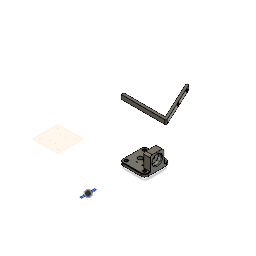
mangaScreenPostMount (Autodesk Fusion 360 design; units mm, degrees)
Autodesk Fusion 360 part; units mm, degrees
sketch "Sketch2" plane through (0, 0, 0) normal (0, 1, 0) x (1, 0, 0)
  circle A0 centre (0, -5) radius 20
  dimension "d26" = 40
  measures "d26" diameter of A0
sketch "Sketch3" plane through (0, 0, 0) normal (0, 1, 0) x (1, 0, 0)
  circle A0 centre (0.421, 74.5094) radius 20
  dimension "d29" = 40
  measures "d29" diameter of A0
sketch "Sketch4" plane through (0, 0, 0) normal (0, 1, 0) x (1, 0, 0)
sketch "Sketch5" plane through (0, 0, 0) normal (0, 1, 0) x (1, 0, 0)
  circle A0 centre (39.3711, 35) radius 20
  dimension "d32" = 40
  measures "d32" diameter of A0
sketch "Sketch6" plane through (0, 0, 0) normal (0, 1, 0) x (1, 0, 0)
sketch "Sketch7" plane through (0, 0, 0) normal (0, 1, 0) x (1, 0, 0)
sketch "Sketch8" plane through (0, 0, 0) normal (0, 1, 0) x (1, 0, 0)
sketch "Sketch9" plane through (0, 0, 0) normal (0, 1, 0) x (1, 0, 0)
sketch "Sketch11" plane through (0, 0, 0) normal (0, 1, 0) x (1, 0, 0)
  line L0 (-185, 0) -> (-64.7091, 0)
  line L1 (-61.9901, 4.2679) -> (-113.6725, 115.1011)
  line L2 (-117.6593, 116.5522) -> (-118.5656, 116.1295)
  line L3 (-185, 0) -> (-185, 5)
  line L4 (-182, 8) -> (-80, 8)
  line L5 (-120.0167, 112.1428) -> (-71.4609, 8.0146)
  line L6 (-80, 8) -> (-71.4609, 8.0146)
  arc A0 (-182, 8) -> (-185, 5) centre (-182, 5) ccw
  arc A1 (-118.5656, 116.1295) -> (-120.0167, 112.1428) centre (-117.2978, 113.4106) ccw
  arc A2 (-113.6725, 115.1011) -> (-117.6593, 116.5522) centre (-116.3914, 113.8332) ccw
  arc A3 (-64.7091, 0) -> (-61.9901, 4.2679) centre (-64.7091, 3) ccw
  dimension "d43" = 65
  dimension "d44" = 130
  dimension "d45" = 7
  dimension "d46" = 8
  dimension "d47" = 3
  dimension "d48" = 3
  dimension "d49" = 3
  dimension "d50" = 3
  measures "d43" angle of L0 L1
  measures "d46" distance of origin
  measures "d47" radius of A0
  measures "d48" radius of A1
  measures "d49" radius of A2
  measures "d50" radius of A3
extrude "Extrude4" add sketch "Sketch11" along normal blind 12 makes body 1
move_body "Move4" bodies 1 to x (1, 0, 0) y (0, 1, 0) z (0, 0, 1) at (70, 0, -150)
hole "Hole5" at (-39.4463, 6, -256.038) direction (-0.906308, 0, 0.422618) diameter 3.8 depth 8 tip angle 180 bodies 1
hole "Hole6" at (-39.4463, 6, -256.038) direction (-0.906308, 0, 0.422618) diameter 7.5 depth 2 tip angle 180 bodies 1
hole "Hole7" at (-45.7905, 6, -253.0797) direction (0.906308, 0, -0.422618) diameter 7.2 depth 4 tip angle 180 bodies 1
hole "Hole8" at (-18.3154, 6, -210.7226) direction (-0.906308, 0, 0.422618) diameter 3.8 depth 8 tip angle 180 bodies 1
hole "Hole9" at (-18.3154, 6, -210.7226) direction (-0.906308, 0, 0.422618) diameter 7.5 depth 2 tip angle 180 bodies 1
hole "Hole10" at (-24.6596, 6, -207.7643) direction (0.906308, 0, -0.422618) diameter 7.2 depth 4 tip angle 180 bodies 1
fillet "Fillet1" radius 0.4 1 edges at (-24.1094, 9.3564, -206.5844) on bodies 1
fillet "Fillet2" radius 0.4 1 edges at (-45.2403, 9.3564, -251.8998) on bodies 1
fillet "Fillet3" radius 0.4 1 edges at (-38.8732, 2.5038, -254.809) on bodies 1
fillet "Fillet4" radius 0.4 1 edges at (-17.7423, 2.5038, -209.4936) on bodies 1
sketch "Sketch12" plane through (0, 0, 0) normal (0, 1, 0) x (1, 0, 0)
  line L0 (-115, 35) -> (-185, 35)
  line L1 (-185, 35) -> (-185, 105)
  line L2 (-185, 105) -> (-115, 105)
  line L3 (-115, 105) -> (-115, 35)
  line L4 (-115, 35) -> (-185, 105) construction
  line L5 (-185, 35) -> (-115, 105) construction
  dimension "d87" = 70
  dimension "d88" = 70
move_body "Move6" bodies 1 to x (1, 0, 0) y (0, 1, 0) z (0, 0, 1) at (-50.7142, 0, -108.7569)
extrude "Extrude5" add sketch "Sketch12" along normal blind 8 separate body makes body 2
hole "Hole11" at (-175, 8, -45) direction (0, -1, 0) diameter 3.8 depth 8 tip angle 180 bodies 2
hole "Hole12" at (-175, 8, -95) direction (0, -1, 0) diameter 3.8 depth 8 tip angle 180 bodies 2
hole "Hole13" at (-125, 8, -45) direction (0, -1, 0) diameter 3.8 depth 8 tip angle 180 bodies 2
hole "Hole14" at (-125, 8, -95) direction (0, -1, 0) diameter 3.8 depth 8 tip angle 180 bodies 2
hole "Hole15" at (-157, 8, -56) direction (0, -1, 0) diameter 2.8 depth 8 tip angle 180 bodies 2
hole "Hole16" at (-157.5, 8, -84) direction (0, -1, 0) diameter 2.8 depth 8 tip angle 180 bodies 2
hole "Hole17" at (-142.5, 8, -56) direction (0, -1, 0) diameter 2.8 depth 8 tip angle 180 bodies 2
hole "Hole18" at (-142.5, 8, -84) direction (0, -1, 0) diameter 2.8 depth 8 tip angle 180 bodies 2
sketch "Sketch13" plane through (0, 0, 0) normal (0, 1, 0) x (1, 0, 0)
sketch "Sketch14" plane through (0, 8, 0) normal (0, 1, 0) x (-1, 0, 0)
  circle A0 centre (142.5, -84) radius 1.4
  circle A1 centre (142.5, -56) radius 1.4
  circle A2 centre (157.5, -84) radius 1.4
  circle A3 centre (157, -56) radius 1.4
  circle A4 centre (125, -95) radius 1.9
  circle A5 centre (125, -45) radius 1.9
  circle A6 centre (175, -95) radius 1.9
  circle A7 centre (175, -45) radius 1.9
  line L0 (115, -105) -> (185, -105)
  line L1 (185, -105) -> (185, -35)
  line L2 (185, -35) -> (115, -35)
  line L3 (115, -35) -> (115, -105)
sketch "Sketch15" plane through (0, 0, 0) normal (0, 1, 0) x (1, 0, 0)
sketch "Sketch16" plane through (0, 0, 0) normal (0, 1, 0) x (1, 0, 0)
move_body "Move7" bodies 2 to x (1, 0, 0) y (0, 1, 0) z (0, 0, 1) at (143.2091, 0.0002, -58.6852)
sketch "Sketch17" plane through (0, 0, 0) normal (0, 1, 0) x (1, 0, 0)
sketch "Sketch18" plane through (0, 0, 0) normal (0, 1, 0) x (1, 0, 0)
hole "Hole19" at (-31.7909, 8.0002, -153.6852) direction (0, -1, 0) diameter 7.2 depth 4 tip angle 180 bodies 2
hole "Hole20" at (18.2091, 8.0002, -153.6852) direction (0, -1, 0) diameter 7.2 depth 4 tip angle 180 bodies 2
hole "Hole21" at (18.2091, 8.0002, -103.6852) direction (0, -1, 0) diameter 7.2 depth 4 tip angle 180 bodies 2
hole "Hole22" at (-31.7909, 8.0002, -103.6852) direction (0, -1, 0) diameter 7.2 depth 4 tip angle 180 bodies 2
move_body "Move8" bodies 2 to x (-1, 0, 0) y (0, -1, 0) z (0, 0, 1) at (-27.5818, 0.0004, 0)
move_body "Move9" bodies 2 to x (1, 0, 0) y (0, 1, 0) z (0, 0, 1) at (0, 13, 0)
hole "Hole23" at (4.2091, 13.0002, -153.6852) direction (0, -1, 0) diameter 7.5 depth 2 tip angle 180 bodies 2
hole "Hole24" at (4.2091, 13.0002, -103.6852) direction (0, -1, 0) diameter 7.5 depth 2 tip angle 180 bodies 2
hole "Hole25" at (-45.7909, 13.0002, -103.6852) direction (0, -1, 0) diameter 7.5 depth 2 tip angle 180 bodies 2
hole "Hole26" at (-45.7909, 13.0002, -153.6852) direction (0, -1, 0) diameter 7.5 depth 2 tip angle 180 bodies 2
move_body "Move10" bodies 2 to x (-1, 0, 0) y (0, -1, 0) z (0, 0, 1) at (8.4182, 22.0004, 0)
hole "Hole27" at (29.2091, 17.0002, -128.6852) direction (0, -1, 0) diameter 6.3 depth 3.5 tip angle 180 bodies 2
sketch "Sketch19" plane through (0, 11.0002, 0) normal (0, -1, 0) x (1, 0, 0)
  circle A0 centre (4.2091, -153.6852) radius 1.9
  circle A1 centre (4.2091, -153.6852) radius 3.75
sketch "Sketch20" plane through (0, 13.5002, 0) normal (0, 1, 0) x (-1, 0, 0)
  circle A0 centre (-29.2091, -128.6852) radius 3.15
sketch "Sketch21" plane through (0, 17.0002, 0) normal (0, 1, 0) x (-1, 0, 0)
  circle A0 centre (-29.2091, -128.6852) radius 3.15
  circle A1 centre (-4.2091, -103.6852) radius 3.6
  circle A2 centre (-54.2091, -103.6852) radius 3.6
  circle A3 centre (-54.2091, -153.6852) radius 3.6
  circle A4 centre (-4.2091, -153.6852) radius 3.6
  circle A5 centre (-36.7091, -142.6852) radius 1.4
  circle A6 centre (-36.7091, -114.6852) radius 1.4
  circle A7 centre (-21.7091, -142.6852) radius 1.4
  circle A8 centre (-22.2091, -114.6852) radius 1.4
  line L0 (-64.2091, -163.6852) -> (5.7909, -163.6852)
  line L1 (5.7909, -163.6852) -> (5.7909, -93.6852)
  line L2 (5.7909, -93.6852) -> (-64.2091, -93.6852)
  line L3 (-64.2091, -93.6852) -> (-64.2091, -163.6852)
  line L4 (-45.1591, -147.7352) -> (-83.2591, -147.7352)
  line L5 (-83.2591, -147.7352) -> (-83.2591, -109.6352)
  line L6 (-83.2591, -109.6352) -> (-45.1591, -109.6352)
  line L7 (-45.1591, -109.6352) -> (-45.1591, -147.7352)
  line L8 (-45.1591, -147.7352) -> (-83.2591, -109.6352) construction
  line L9 (-83.2591, -147.7352) -> (-45.1591, -109.6352) construction
  dimension "d195" = 38.1
  dimension "d196" = 38.1
extrude "Extrude6" add sketch "Sketch21" along normal blind 38.1 contours L3 L4 L6 L7 bodies 2
sketch "Sketch22" plane through (0, 0, 0) normal (0, 1, 0) x (1, 0, 0)
sketch "Sketch23" plane through (0, 0, 0) normal (0, 1, 0) x (1, 0, 0)
  line L0 (11, 10) -> (15, 10)
  line L1 (15, 10) -> (15, -30)
  line L2 (15, -30) -> (11, -30)
  line L3 (11, -30) -> (11, 10)
  line L4 (11, 10) -> (15, -30) construction
  line L5 (15, 10) -> (11, -30) construction
  dimension "d177" = 40
  dimension "d178" = 4
hole "Hole28" at (-142.7142, 6, -266.7569) direction (0, 0, 1) diameter 8.2 depth 3 tip angle 180 bodies 1
hole "Hole29" at (-102.7142, 6, -266.7569) direction (0, 0, 1) diameter 8.2 depth 3 tip angle 180 bodies 1
fillet "Fillet5" radius 0.5 1 edges at (-138.8916, 7.4826, -266.7569) on bodies 1
fillet "Fillet6" radius 0.5 1 edges at (-98.8916, 7.4826, -266.7569) on bodies 1
fillet "Fillet7" radius 10 1 edges at (64.2091, 13.0002, -93.6852) on bodies 2
sketch "Sketch24" plane through (0, 0, 0) normal (0, 1, 0) x (1, 0, 0)
fillet "Fillet8" radius 10 1 edges at (-5.7909, 13.0002, -93.6852) on bodies 2
fillet "Fillet9" radius 10 1 edges at (-5.7909, 13.0002, -163.6852) on bodies 2
fillet "Fillet10" radius 10 1 edges at (64.2091, 13.0002, -163.6852) on bodies 2
fillet "Fillet11" radius 1 1 edges at (5.5109, 17.0002, -107.0416) on bodies 2
fillet "Fillet12" radius 1 1 edges at (5.5109, 17.0002, -157.0416) on bodies 2
fillet "Fillet13" radius 1 1 edges at (55.5109, 17.0002, -157.0416) on bodies 2
fillet "Fillet14" radius 1 1 edges at (55.5109, 17.0002, -107.0416) on bodies 2
fillet "Fillet15" radius 5 1 edges at (54.6841, 55.1002, -109.6352) on bodies 2
fillet "Fillet16" radius 5 1 edges at (54.6841, 55.1002, -147.7352) on bodies 2
hole "Hole30" at (64.2091, 36.0502, -128.6852) direction (-1, 0, 0) diameter 25.6 depth 10 tip angle 180 bodies 2
fillet "Fillet17" radius 2 1 edges at (64.2091, 24.1164, -124.0565) on bodies 2
hole "Hole31" at (45.1591, 36.0502, -128.6852) direction (1, 0, 0) diameter 6.3 depth 25.4 tip angle 180 bodies 2
hole "Hole32" at (45.1591, 36.0502, -128.6852) direction (1, 0, 0) diameter 10.2 depth 6 tip angle 180 bodies 2
fillet "Fillet18" radius 1 1 edges at (45.1591, 40.8051, -126.841) on bodies 2
fillet "Fillet19" radius 0.8 1 edges at (2.853, 9.0002, -157.1814) on bodies 2
fillet "Fillet20" radius 0.8 1 edges at (2.853, 9.0002, -107.1814) on bodies 2
fillet "Fillet21" radius 0.8 1 edges at (52.853, 9.0002, -107.1814) on bodies 2
fillet "Fillet22" radius 0.8 1 edges at (52.853, 9.0002, -157.1814) on bodies 2
fillet "Fillet23" radius 1 9 edges at (64.2091, 17.0002, -150.7102) (61.2801, 17.0002, -160.7563) (29.2091, 17.0002, -163.6852) (-2.862, 17.0002, -160.7563) (-5.7909, 17.0002, -128.6852) (-2.862, 17.0002, -96.6141) (29.2091, 17.0002, -93.6852) (61.2801, 17.0002, -96.6141) (64.2091, 17.0002, -106.6602) on bodies 2
fillet "Fillet24" radius 1 5 edges at (45.1591, 33.5502, -109.6352) (45.1591, 53.6357, -111.0997) (45.1591, 55.1002, -128.6852) (45.1591, 53.6357, -146.2708) (45.1591, 33.5502, -147.7352) on bodies 2
sketch "Sketch25" plane through (45.1591, 0, 0) normal (-1, 0, 0) x (0, 0, 1)
  line L0 (-146.7352, 50.1002) -> (-146.7352, 17.0002)
  line L1 (-146.7352, 17.0002) -> (-110.6352, 17.0002)
  line L2 (-110.6352, 17.0002) -> (-110.6352, 50.1002)
  arc A0 (-110.6352, 50.1002) -> (-114.6352, 54.1002) centre (-114.6352, 50.1002) ccw
  line L3 (-114.6352, 54.1002) -> (-142.7352, 54.1002)
  arc A1 (-142.7352, 54.1002) -> (-146.7352, 50.1002) centre (-142.7352, 50.1002) ccw
  circle A2 centre (-128.6852, 36.0502) radius 6.1
sketch "Sketch26" plane through (0, 0, 0) normal (1, 0, 0) x (0, 0, -1)
sketch "Sketch27" plane through (0, 17.0002, 0) normal (0, 1, 0) x (-1, 0, 0)
  line L0 (-63.2091, -103.6852) -> (-63.2091, -109.6352)
  line L1 (-63.2091, -109.6352) -> (-46.1591, -109.6352)
  arc A0 (-45.1591, -110.6352) -> (-46.1591, -109.6352) centre (-46.1591, -110.6352) ccw
  line L2 (-45.1591, -110.6352) -> (-45.1591, -146.7352)
  arc A1 (-46.1591, -147.7352) -> (-45.1591, -146.7352) centre (-46.1591, -146.7352) ccw
  line L3 (-46.1591, -147.7352) -> (-63.2091, -147.7352)
  line L4 (-63.2091, -147.7352) -> (-63.2091, -153.6852)
  arc A2 (-63.2091, -153.6852) -> (-54.2091, -162.6852) centre (-54.2091, -153.6852) ccw
  line L5 (-54.2091, -162.6852) -> (-4.2091, -162.6852)
  arc A3 (-4.2091, -162.6852) -> (4.7909, -153.6852) centre (-4.2091, -153.6852) ccw
  line L6 (4.7909, -153.6852) -> (4.7909, -103.6852)
  arc A4 (4.7909, -103.6852) -> (-4.2091, -94.6852) centre (-4.2091, -103.6852) ccw
  line L7 (-4.2091, -94.6852) -> (-54.2091, -94.6852)
  arc A5 (-54.2091, -94.6852) -> (-63.2091, -103.6852) centre (-54.2091, -103.6852) ccw
  circle A6 centre (-54.2091, -153.6852) radius 4.6
  circle A7 centre (-4.2091, -103.6852) radius 4.6
  circle A8 centre (-29.2091, -128.6852) radius 3.15
  circle A9 centre (-36.7091, -142.6852) radius 1.4
  circle A10 centre (-36.7091, -114.6852) radius 1.4
  circle A11 centre (-21.7091, -142.6852) radius 1.4
  circle A12 centre (-22.2091, -114.6852) radius 1.4
  circle A13 centre (-4.2091, -153.6852) radius 4.6
  circle A14 centre (-54.2091, -103.6852) radius 4.6
  circle A15 centre (-17.4511, -128.6852) radius 6
  dimension "d229" = 12
  measures "d229" diameter of A15
extrude "Extrude7" cut sketch "Sketch27" against normal blind 12 contours A15 bodies 2
